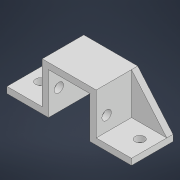
# Autodesk Inventor part: Horizontal Support Bracket
Saved by Autodesk Inventor 2022 (Build 260153000, 153)
## iProperties
Created: 2023-01-13
Part Number: Horizontal Support Bracket
Material: Generic
Document SubType Name: Modeling
Designer: Ryan Mitcham
Density: 1 g/cm^3
Appearance: Default
Author: Ryan Mitcham
Autodesk Inventor part; units mm, degrees
ref_plane "YZ Plane" through (0, 0, 0) normal (1, 0, 0) x (0, 1, 0)
ref_plane "XZ Plane" through (0, 0, 0) normal (0, 1, 0) x (-1, 0, 0)
ref_plane "XY Plane" through (0, 0, 0) normal (0, 0, 1) x (1, 0, 0)
sketch "Sketch2" plane through (0, 0, 0) normal (0, 0, 1) x (1, 0, 0)
  line L0 (-30, 11.5) -> (-30, -11.5)
  line L1 (-30, -11.5) -> (-10, -11.5)
  line L2 (-10, -11.5) -> (-10, 8.5)
  line L3 (-10, 8.5) -> (10, 8.5)
  line L4 (10, 8.5) -> (10, -11.5)
  line L5 (10, -11.5) -> (30, -11.5)
  line L6 (30, -11.5) -> (30, 11.5)
  line L7 (30, 11.5) -> (-30, 11.5)
  point P0 (0, 0)
  point P1 (0, 11.5)
  point P2 (30, 0)
  dimension "d6" = 23
  dimension "d7" = 20
  dimension "d8" = 20
  constraints: 16 end point, 7 perpendicular, 3 equal length, 2 midpoint, 1 horizontal alignment, 1 vertical, 1 vertical alignment
  measures "d6" distance of L5.end L6.end
  measures "d7" distance of L4.end L5.end
  measures "d8" distance of L2.end L3.end
extrude "Extrusion1" add sketch "Sketch2" along normal blind 3
sketch "Sketch3" plane through (0, 0, 3) normal (0, 0, 1) x (1, 0, 0)
  line L0 (30, 11.5) -> (-30, 11.5) projected
  line L1 (-13, 11.5) -> (-30, -8.5)
  line L2 (-30, 11.5) -> (-30, -11.5) projected
  line L3 (-30, 11.5) -> (-13, 11.5)
  line L4 (-10, -11.5) -> (-10, 8.5) projected
  line L5 (13, 11.5) -> (30, -8.5)
  line L6 (30, -11.5) -> (30, 11.5) projected
  line L7 (10, 8.5) -> (10, -11.5) projected
  line L8 (10, -11.5) -> (30, -11.5) projected
  point P0 (0, 0)
  dimension "d11" = 3
  dimension "d12" = 3
  dimension "d13" = 3
  dimension "d14" = 3
  constraints: 6 end point, 4 point on line, 1 horizontal
  measures "d11" distance of L2.end L1.end
  measures "d12" distance from line of L1.start L4
  measures "d13" distance from line of L7 L5.start
  measures "d14" distance from line of L8 L5.end
extrude "Extrusion2" cut sketch "Sketch3" against normal through all
sketch "Sketch4" plane through (0, 0, 3) normal (0, 0, 1) x (1, 0, 0)
  line L0 (-30, -8.5) -> (-30, -11.5) projected
  line L1 (-30, -8.5) -> (-13, -8.5)
  line L2 (13, 11.5) -> (-13, 11.5) projected
  line L3 (-13, -8.5) -> (-13, 11.5)
  line L4 (30, -11.5) -> (30, -8.5) projected
  line L5 (30, -8.5) -> (13, -8.5)
  line L6 (13, -8.5) -> (13, 11.5)
  line L7 (30, -8.5) -> (13, 11.5) projected
  line L8 (13, 11.5) -> (-13, 11.5) projected
  line L9 (-13, 11.5) -> (-30, -8.5) projected
  line L10 (-30, -8.5) -> (-30, -11.5) projected
  line L11 (-30, -11.5) -> (-10, -11.5) projected
  line L12 (-10, -11.5) -> (-10, 8.5) projected
  line L13 (-10, 8.5) -> (10, 8.5) projected
  line L14 (10, 8.5) -> (10, -11.5) projected
  line L15 (10, -11.5) -> (30, -11.5) projected
  line L16 (30, -11.5) -> (30, -8.5) projected
  point P0 (0, 0)
  dimension "d17" = 90
  dimension "d20" = 90
  constraints: 8 end point, 2 horizontal
  measures "d17" angle of L1 L3
  measures "d20" angle of L5 L6
extrude "Extrusion3" add sketch "Sketch4" along normal blind 17 contours L1 L3 L2 L6 L5 L4 L15 L14 L13 L12 L11 L0
sketch "Sketch5" plane through (-13, -8.5, 3) normal (-1, 0, 0) x (0, 0, 1)
  line L0 (-3, 17) -> (17, 17) projected
  line L1 (17, 20) -> (17, 0) projected
  point P0 (-3, 8.5)
  point P1 (12, 7)
  dimension "d23" = 10
  dimension "d24" = 5
  measures "d23" distance from line of point (12, 7) L0
  measures "d24" distance from line of L1 point (12, 7)
hole "Hole1" at (-13, -1.5, 15) direction (1, 0, 0) diameter 4.5 end through all
sketch "Sketch6" plane through (-30, -8.5, 3) normal (0, 1, 0) x (1, 0, 0)
  line L0 (17, -17) -> (0, -17) projected
  line L1 (0, 0) -> (0, -17) projected
  line L2 (60, 0) -> (60, -17) projected
  point P0 (30, 3)
  point P1 (6, -7)
  point P2 (54, -7)
  dimension "d32" = 10
  dimension "d33" = 6
  dimension "d34" = 6
  constraints: 1 horizontal alignment
  measures "d32" distance from line of point (6, -7) L0
  measures "d33" distance from line of L1 point (6, -7)
  measures "d34" distance from line of L2 point (54, -7)
hole "Hole2" at (-24, -8.5, 10) at (24, -8.5, 10) direction (0, -1, 0) diameter 4.5 end through all
equation "\"d34\" = d33"
body "Solid1"
